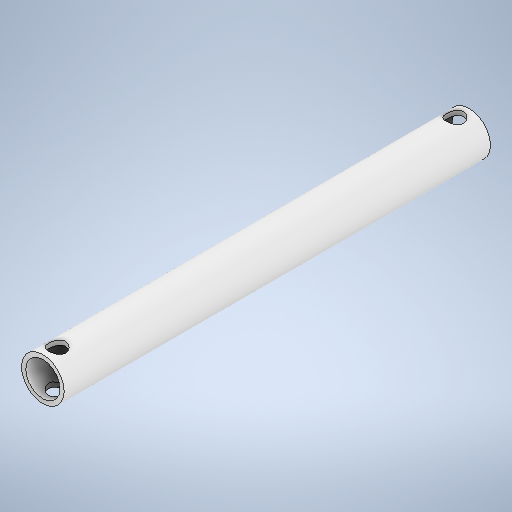
# Autodesk Inventor part: Shifter Post
Saved by Autodesk Inventor 2025.2 (Build 292293000, 293)
## iProperties
Created: 2025-02-09
Part Number: Shifter Post
Material: PVC-Piping
Document SubType Name: Modeling
Designer: eason
Density: 1.4 g/cm^3
Appearance: Smooth - White
Author: eason
Autodesk Inventor part; units mm, degrees
ref_plane "YZ Plane" through (0, 0, 0) normal (1, 0, 0) x (0, 1, 0)
ref_plane "XY Plane" through (0, 0, 0) normal (0, 0, 1) x (1, 0, 0)
sketch "Sketch1" plane through (0, 0, 0) normal (0, 0, 1) x (1, 0, 0)
  circle A0 centre (0, 0) radius 7.5
  circle A1 centre (0, 0) radius 6
  dimension "d0" = 15
  dimension "d1" = 12
  constraints: 2 centre point, 2 coincident
  measures "d0" diameter of A0
  measures "d1" diameter of A1
extrude "Extrusion1" add sketch "Sketch1" along normal blind 150
ref_plane "Work Plane1" through (0, -7.5, 0) normal (0, 1, 0) x (-1, 0, 0)
sketch "Sketch2" plane through (0, -7.5, 0) normal (0, 1, 0) x (-1, 0, 0)
  circle A0 centre (0, 5) radius 3
  line L0 (0, -30) -> (0, 180) projected
  line L1 (7.5, 0) -> (-7.5, 0) projected
  circle A1 centre (0, 145) radius 3
  line L2 (7.5, 150) -> (-7.5, 150) projected
  point P0 (0, 0)
  dimension "d4" = 6
  dimension "d5" = 5
  dimension "d8" = 6
  dimension "d9" = 5
  constraints: 2 centre point, 2 point on line
  measures "d4" diameter of A0
  measures "d5" distance from line of L1 A0.centre
  measures "d8" diameter of A1
  measures "d9" distance from line of A1.centre L2
extrude "Extrusion2" cut sketch "Sketch2" along normal through all
body "Solid1"
